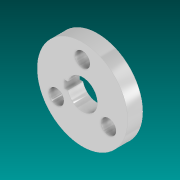
# Autodesk Inventor part: spiebaanplaatKlein
Saved by Autodesk Inventor 2020.3 (Build 243373000, 373)
## iProperties
Created: 2020-05-24
Part Number: spiebaanplaatKlein
Material: Aluminum 6061
Document SubType Name: Modeling
Designer: Svend
Density: 2.7 g/cm^3
Appearance: Aluminum - Polished
Author: Svend
Autodesk Inventor part; units mm, degrees
ref_plane "YZ Plane" through (0, 0, 0) normal (1, 0, 0) x (0, 1, 0)
ref_plane "XZ Plane" through (0, 0, 0) normal (0, 1, 0) x (-1, 0, 0)
ref_plane "Work Plane1" through (0, 0, 0) normal (0, 0, 1) x (1, 0, 0)
sketch "Sketch1" plane through (0, 0, 0) normal (0, 0, 1) x (1, 0, 0)
  circle A0 centre (0, 0) radius 12 projected
  circle A1 centre (-6.9282, -4) radius 2 projected
  circle A2 centre (6.9282, -4) radius 2 projected
  circle A3 centre (0, 8) radius 2 projected
  line L0 (-4.8, 1) -> (-4.8, -1) projected
  line L1 (-3.873, 1) -> (-4.8, 1) projected
  arc A4 (-3.873, -1) -> (-3.873, 1) centre (0, 0) ccw projected
  line L2 (-4.8, -1) -> (-3.873, -1) projected
  point P0 (0, 0)
extrude "Extrusion1" add sketch "Sketch1" along normal blind 4 contours A0 | A1 | A2 | A3
sketch "Sketch2" plane through (0, 0, 0) normal (0, 0, -1) x (-1, 0, 0)
  point P0 (0, 0)
  point P1 (-6.9282, -4)
  point P2 (0, 8)
  point P3 (6.9282, -4)
hole "Hole1" at (6.9282, -4, 0) at (0, 8, 0) at (-6.9282, -4, 0) direction (0, 0, 1) diameter 4 end through all clearance for "Countersunk Flat Head Screw ISO 2009/7046" size "M4" standard "ISO"
body "Solid1"
